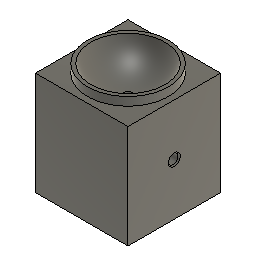
floating_ball_fixture_25.4mm (Autodesk Fusion 360 design; units mm, degrees)
Autodesk Fusion 360 part; units mm, degrees
imported_body "Base Feature1" makes body 1
sketch "bottom" plane through (0, 0, 0) normal (0, 0, 1) x (1, 0, 0)
  line L0 (16.56, -16.56) -> (-16.56, -16.56)
  line L1 (-16.56, -16.56) -> (-16.56, 16.56)
  line L2 (-16.56, 16.56) -> (16.56, 16.56)
  line L3 (16.56, 16.56) -> (16.56, -16.56)
  line L4 (16.56, -16.56) -> (-16.56, 16.56) construction
  line L5 (-16.56, -16.56) -> (16.56, 16.56) construction
  circle A0 centre (0, 0) radius 13.97
  circle A1 centre (0, 0) radius 2.705
  circle A2 centre (0, 0) radius 1.473
  dimension "d2" = 33.12
  dimension "d4" = 27.94
  dimension "d15" = 5.41
  dimension "d20" = 2.946
  constraint horizontal L0
  constraint perpendicular L0 L1
  constraint parallel L0 L2
  constraint parallel L1 L3
  constraint coincident L4 A0.centre
  constraint coincident L5 A0.centre
  constraint coincident A0.centre A1.centre
  constraint equal L1 L2
  measures "d2" distance of L1.end L2.end
  measures "d4" diameter of A0
  measures "d15" diameter of A1
  measures "d20" diameter of A2
extrude "Extrude3" add sketch "bottom" along normal blind 14 separate body contours A1 | A2 makes body 2
extrude "Extrude2" add sketch "bottom" along normal blind 40 separate body contours A0 | A1 | A2 makes body 3
extrude "Extrude1" add sketch "bottom" along normal blind 37 separate body contours L0 L1 L2 L3 | A0 | A1 | A2 makes body 4
combine "Combine1" operation add target body 3 tool bodies 4
combine "Combine2" operation cut target body 3 tool bodies 2
chamfer "Chamfer1" distance 0.4 angle 45 1 edges at (-2.5219, -0.9782, 0) on bodies 3
extrude "Extrude4" cut sketch "bottom" along normal blind 40 contours A2 bodies 3
ref_plane "WorkPlane1" through (16.56, 0, 18.5) normal (1, 0, 0) x (0, 1, 0)
sketch "side" plane through (16.56, 0, 18.5) normal (1, 0, 0) x (0, 0, -1)
  line L0 (0, 0) -> (18.5, 0) construction
  circle A0 centre (0, 0) radius 1.727
  dimension "d25" = 18.5
  dimension "d26" = 3.454
  constraint coincident L0.start A0.centre
  constraint horizontal L0
  measures "d25" distance of L0.start L0.end
  measures "d26" diameter of A0
extrude "Extrude5" cut sketch "side" against normal blind 5.5 bodies 3
chamfer "Chamfer2" distance 0.4 angle 45 1 edges at (16.56, 0.6245, 20.1101) on bodies 3
sphere "SpherePrimitive2" add diameter 27.6 placed x (-1, 0, 0) y (0, -1, 0) z (0, 0, 1) at (0, 0, 40) separate body makes body 5
move_body "Move3" bodies 5 to x (1, 0, 0) y (0, 1, 0) z (0, 0, 1) at (0, 0, 4.0278)
combine "Combine4" operation cut target body 3 tool bodies 5
move_face "OffsetFaces1" offset 0.5 1 faces at (13.9006, -1.391, 39) on bodies 3
hidden bodies 1
equation "width_length = ball_cutout_dia * 1.2"
equation "d2 = width_length"
equation "ball_dia = 25.4 mm"
equation "d4 = ball_dia * 1.1"
equation "height = 37 mm"
equation "d6 = height"
equation "lip_height = 3 mm"
equation "d9 = height + lip_height"
equation "tap_quarter_28_dia = 2.705 mm * 2"
equation "tap_8_32_dia = 1.727 mm * 2"
equation "bottom_hole_depth = 14 mm"
equation "top_hole_dia = 1.473 mm * 2"
equation "d15 = tap_quarter_28_dia"
equation "d16 = bottom_hole_depth"
equation "chamfer = 0.4 mm"
equation "d19 = chamfer"
equation "d20 = top_hole_dia"
equation "side_hole_depth = 5.5 mm"
equation "d25 = height / 2"
equation "d26 = tap_8_32_dia"
equation "d27 = -side_hole_depth"
equation "d29 = chamfer"
equation "ball_cutout_dia = ball_dia + 2.2 mm"
equation "d33 = ball_cutout_dia"
equation "ball_cut_height_offset = ball_cutout_dia * 0.15"
named bodies: "original", "main", "sphere"
